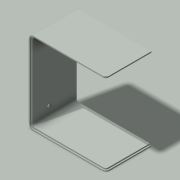
# Autodesk Inventor part: SimpleFrontRightPlate
Saved by Autodesk Inventor 2015 (Build 190159000, 159)
## iProperties
Created: 2015-07-12
Part Number: SimpleFrontRightPlate
Material: Generic
Document SubType Name: Modeling
Designer: -
Density: 1 g/cm^3
Appearance: Default
Author: -
Autodesk Inventor part; units mm, degrees
ref_plane "YZ Plane" through (0, 0, 0) normal (1, 0, 0) x (0, 1, 0)
ref_plane "XZ Plane" through (0, 0, 0) normal (0, 1, 0) x (-1, 0, 0)
ref_plane "XY Plane" through (0, 0, 0) normal (0, 0, 1) x (1, 0, 0)
ref_plane "Work Plane1" through (0, 0, 0) normal (0, 0, 1) x (1, 0, 0)
sketch "Sketch1" plane through (0, 0, 0) normal (0, 0, 1) x (1, 0, 0)
  arc A0 (-24.0847, -30.575) -> (-20.0847, -34.575) centre (-20.0847, -30.575) ccw projected
  line L0 (-20.0847, -34.575) -> (40.4221, -34.575) projected
  line L1 (40.4221, -34.575) -> (40.4221, -30.575) projected
  line L2 (40.4221, -30.575) -> (-16.0847, -30.575) projected
  arc A1 (-20.0847, -26.575) -> (-16.0847, -30.575) centre (-16.0847, -26.575) ccw projected
  line L3 (-20.0847, -26.575) -> (-20.0847, -27.765) projected
  line L4 (-20.0847, -27.765) -> (-22.0847, -27.765) projected
  line L5 (-22.0847, -27.765) -> (-22.0847, -21.765) projected
  line L6 (-22.0847, -21.765) -> (-20.0847, -21.765) projected
  line L7 (-20.0847, -21.765) -> (-20.0847, 21.765) projected
  line L8 (-20.0847, 21.765) -> (-22.0847, 21.765) projected
  line L9 (-22.0847, 21.765) -> (-22.0847, 27.765) projected
  line L10 (-22.0847, 27.765) -> (-20.0847, 27.765) projected
  line L11 (-20.0847, 27.765) -> (-20.0847, 26.575) projected
  arc A2 (-16.0847, 30.575) -> (-20.0847, 26.575) centre (-16.0847, 26.575) ccw projected
  line L12 (-16.0847, 30.575) -> (40.4221, 30.575) projected
  line L13 (40.4221, 30.575) -> (40.4221, 34.575) projected
  line L14 (40.4221, 34.575) -> (-20.0847, 34.575) projected
  arc A3 (-20.0847, 34.575) -> (-24.0847, 30.575) centre (-20.0847, 30.575) ccw projected
  line L15 (-24.0847, 30.575) -> (-24.0847, -30.575) projected
  line L16 (40.4221, -34.575) -> (-20.0847, -34.575)
  line L17 (-24.0847, -30.575) -> (-24.0847, 30.575)
  line L18 (-20.0847, 34.575) -> (40.4221, 34.575)
  line L19 (40.4221, 32.575) -> (-20.0847, 32.575)
  line L20 (-22.0847, 30.575) -> (-22.0847, -30.575)
  line L21 (-20.0847, -32.575) -> (40.4221, -32.575)
  arc A4 (-20.0847, 32.575) -> (-22.0847, 30.575) centre (-20.0847, 30.575) ccw
  arc A5 (-22.0847, -30.575) -> (-20.0847, -32.575) centre (-20.0847, -30.575) ccw
  arc A6 (-24.0847, -30.575) -> (-20.0847, -34.575) centre (-20.0847, -30.575) ccw
  arc A7 (-20.0847, 34.575) -> (-24.0847, 30.575) centre (-20.0847, 30.575) ccw
  point P0 (0, 0)
  dimension "d0" = 2
  dimension "d1" = 4
  constraints: 12 end point, 8 point on circle, 8 tangent, 4 centre point, 3 parallel, 2 equal radius, 2 midpoint, 1 collinear, 1 perpendicular
  measures "d0" radius of A4
  measures "d1" radius of A6
extrude "Extrusion1" add sketch "Sketch1" along normal blind 37 contours L15 A3 L14 L13 L19 A4 L20 L9 L5 A5 L21 L1 L0 A0
lip "Lip1" kind lip height 1 width 1 edges at (-22.9131, 33.4034, 37) (-24.0847, 0, 37) (-22.9131, -33.4034, 37) (10.1687, -34.575, 37) (10.1687, 34.575, 37) guide face at (-22.7513, -10.1917, 37)
lip "Lip4" kind groove height 1 width 1 edges at (40.4221, -32.575, 18.5) guide face at (40.4221, -33.575, 12.3333)
lip "Lip5" kind groove height 1 width 1 edges at (40.4221, 32.575, 18.5) guide face at (40.4221, 33.575, 12.3333)
fillet "Fillet1" radius 2 2 edges at (39.4221, -33.075, 37) (39.4221, 33.075, 37)
fillet "Fillet4" radius 3 2 edges at (40.4221, 34.075, 38) (40.4221, -34.075, 38)
sketch "Sketch2" plane through (-24.0847, -30.575, 0) normal (-1, 0, 0) x (0, 0, 1)
  circle A0 centre (22.895, 55.34) radius 1.4 projected
  circle A1 centre (22.895, 5.81) radius 1.4 projected
  point P0 (0, 30.575)
extrude "Extrusion2" cut sketch "Sketch2" against normal blind 10
chamfer "Chamfer1" distance 1 angle 45 2 edges at (-24.0847, 24.765, 21.495) (-24.0847, -24.765, 21.495)
body "Solid1"
